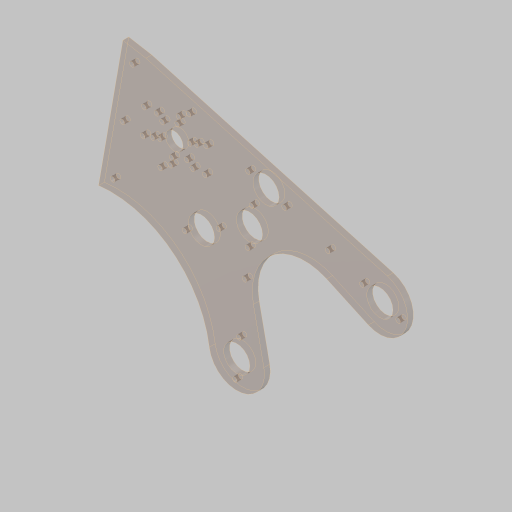
# Autodesk Inventor part: GP7-001
Saved by Autodesk Inventor 2023.5 (Build 275446000, 446)
## iProperties
Created: 2025-02-24
Part Number: GP7-001
Material: Polycarbonate, Smoke
Document SubType Name: Modeling
Designer: dlangdon
Density: 1.2 g/cm^3
Appearance: Polycarbonate - Smoked
Author: dlangdon
Autodesk Inventor part; units mm, degrees
ref_plane "YZ Plane" through (0, 0, 0) normal (1, 0, 0) x (0, 1, 0)
ref_plane "XZ Plane" through (0, 0, 0) normal (0, 1, 0) x (-1, 0, 0)
ref_plane "XY Plane" through (0, 0, 0) normal (0, 0, 1) x (1, 0, 0)
sketch "Sketch1" plane through (0, 0, 0) normal (0, 0, 1) x (1, 0, 0)
  circle A0 centre (77.8301, 65.3072) radius 50.8 construction
  circle A1 centre (-77.8301, -65.3072) radius 50.8 construction
  circle A2 centre (0, 0) radius 50.8 construction
  line L0 (-38.9151, -32.6536) -> (38.9151, 32.6536) construction
  line L1 (77.8301, 65.3072) -> (-77.8301, -65.3072) construction
  line L2 (-3.81, 6.5991) -> (-3.81, 50.6569) construction
  line L3 (-409.5487, -116.1072) -> (455.8434, -116.1072) construction
  circle A3 centre (141.8525, -58.9572) radius 57.15 construction
  circle A4 centre (77.8301, 65.3072) radius 14.2621
  circle A5 centre (-77.8301, -65.3072) radius 14.2621
  circle A6 centre (-3.81, 6.5991) radius 57.15 construction
  circle A7 centre (-77.8301, -65.3072) radius 30.1371 construction
  circle A8 centre (77.8301, 65.3072) radius 30.1371 construction
  circle A9 centre (-46.054, 109.6985) radius 14.2621
  line L4 (-46.054, 109.6985) -> (77.8301, 65.3072) construction
  circle A10 centre (77.8301, 65.3072) radius 14.2875 construction
  circle A11 centre (-77.8301, -65.3072) radius 14.2875 construction
  circle A12 centre (-64.0611, 65.5679) radius 14.2621
  line L5 (-77.8301, -65.3072) -> (-64.0611, 65.5679) construction
  circle A13 centre (-64.0611, 65.5679) radius 23.8316 construction
  circle A14 centre (-46.054, 109.6985) radius 23.8316 construction
  line L6 (19.8995, 58.5989) -> (65.3273, 37.886)
  line L7 (-48.3441, -59.0766) -> (-59.7253, -5.2163)
  arc A15 (19.8995, 58.5989) -> (-59.7253, -5.2163) centre (-3.81, 6.5991) ccw
  line L8 (-201.688, 172.6254) -> (-176.6739, 168.2148)
  line L9 (-176.6739, 168.2148) -> (-203.1379, 18.1301) construction
  line L10 (-203.1379, 18.1301) -> (-228.152, 22.5407) construction
  line L11 (-228.152, 22.5407) -> (-201.688, 172.6254) construction
  line L12 (-247.4634, -86.98) -> (29.0821, -135.7424) construction
  line L13 (-202.7907, 166.3719) -> (190.615, 97.0039) construction
  line L14 (-202.7907, 166.3719) -> (-247.4634, -86.98) construction
  circle A16 centre (-145.793, 105.6556) radius 31.75 construction
  line L15 (-66.5546, 41.8671) -> (-72.5149, -14.786) construction
  circle A17 centre (21.0409, 85.6565) radius 9.525 construction
  line L16 (-189.1809, 170.4201) -> (-215.6449, 20.3354) construction
  line L17 (-191.9376, 154.7863) -> (-212.8883, 35.9692) construction
  circle A18 centre (-145.793, 105.6556) radius 17.4625 construction
  circle A19 centre (-145.793, 105.6556) radius 9.525
  circle A20 centre (-46.054, 109.6985) radius 30.1816 construction
  line L18 (-201.688, 172.6254) -> (-228.152, 22.5407)
  arc A21 (65.3273, 37.886) -> (85.9918, 94.3181) centre (77.8301, 65.3072) ccw
  arc A22 (-107.6731, -69.5072) -> (-48.3441, -59.0766) centre (-77.8301, -65.3072) ccw
  line L19 (-145.793, 105.6556) -> (-129.3836, 111.6281) construction
  line L20 (-111.4825, 118.1436) -> (-180.1035, 93.1676) construction
  circle A23 centre (-180.1035, 93.1676) radius 4.7625 construction
  line L21 (0, 0) -> (-3.81, 6.5991) construction
  circle A24 centre (77.8301, 65.3072) radius 28.6512 construction
  line L22 (65.2741, 39.5538) -> (-52.3042, 96.8789) construction
  line L23 (84.4878, 93.1742) -> (-42.7399, 123.5703) construction
  line L24 (-176.6739, 168.2148) -> (85.9918, 94.3181)
  line L25 (-145.793, 105.6556) -> (-116.2701, 36.6349) construction
  circle A25 centre (-116.2701, 36.6349) radius 31.75 construction
  circle A26 centre (-116.2701, 36.6349) radius 14.2621
  line L26 (-64.0611, 65.5679) -> (-116.2701, 36.6349) construction
  circle A27 centre (-145.793, 105.6556) radius 25.4 construction
  arc A28 (-107.6731, -69.5072) -> (-228.152, 22.5407) centre (-214.5697, -84.5514) ccw
  circle A29 centre (-145.793, 105.6556) radius 36.5125 construction
  line L27 (-178.8846, 121.0865) -> (-145.793, 105.6556) construction
  point P0 (-69.5348, 13.5405)
  point P1 (-202.4129, 95.3778)
  point P2 (-202.4129, 95.3778)
  point P3 (-142.7607, 122.8528)
  point P4 (-159.1701, 116.8803)
  point P5 (-162.2024, 99.6831)
  point P6 (-148.8254, 88.4584)
  point P7 (-132.416, 94.4309)
  point P8 (-121.9248, 114.3429)
  point P9 (-141.3824, 130.6697)
  point P10 (-165.2505, 121.9824)
  point P11 (-169.6612, 96.9683)
  point P12 (-150.2037, 80.6415)
  point P13 (-126.3355, 89.3288)
  point P14 (-158.281, 139.9661)
  point P15 (-180.1035, 93.1676)
  point P16 (-133.305, 71.3451)
  point P17 (-130.3622, 138.7472)
  point P18 (-161.2239, 72.564)
  point P19 (-112.7015, 90.2248)
  dimension "d7" = 101.6
  dimension "d18" = 47.6631
  dimension "d34" = 34.925
  dimension "d65" = 50.8
  dimension "d3" = 50
  dimension "d4" = 0
  dimension "d8" = 101.6
  dimension "d9" = 28.5242
  dimension "d10" = 101.6
  dimension "d11" = 114.3
  dimension "d12" = 114.3
  dimension "d13" = 15.875
  dimension "d14" = 15.875
  dimension "d15" = 131.5974
  dimension "d16" = 28.575
  dimension "d17" = 131.5974
  dimension "d19" = 47.6631
  dimension "d22" = 25.4
  dimension "d23" = 152.4
  dimension "d26" = 257.2602
  dimension "d27" = 63.5
  dimension "d30" = 203.2
  dimension "d31" = 10
  dimension "d32" = 19.05
  dimension "d33" = 120.65
  dimension "d35" = 19.05
  dimension "d36" = 6.35
  dimension "d40" = 360
  dimension "d44" = 9.525
  dimension "d55" = 80
  dimension "d56" = 7.62
  dimension "d58" = 57.3024
  dimension "d59" = 63.5
  dimension "d60" = 75.0697
  dimension "d61" = 59.69
  dimension "d62" = 55
  dimension "d68" = 360
  dimension "d70" = 41.275
  dimension "d71" = 60
  dimension "d82" = 360
  dimension "d87" = 360
  dimension "d89" = 45
  dimension "d90" = 6.35
  dimension "d91" = 20.955
  dimension "d92" = 107.95
  constraints: 56 end point, 26 centre point, 24 coincident, 23 point on circle, 14 tangent, 7 midpoint, 6 equal radius, 5 point on line, 4 collinear, 4 parallel, 2 horizontal, 1 concentric, 1 perpendicular, 1 vertical, 39 other
  measures "d3" angle of L2 L0
  measures "d4" distance between parallel lines of L0 L1
  measures "d8" diameter of A2
  measures "d9" diameter of A4
  measures "d10" diameter of A0
  measures "d11" diameter of A3
  measures "d12" diameter of A6
  measures "d13" radial gap between concentric circles of A5 A7
  measures "d14" radial gap between concentric circles of A4 A8
  measures "d15" distance of L4.start L4.end
  measures "d16" diameter of A10
  measures "d17" distance of L5.start L5.end
  measures "d19" diameter of A14
  measures "d22" distance of L9.end L10.end
  measures "d23" distance of L10.end L8.start
  measures "d26" distance of L13.start L12.start
  measures "d27" diameter of A16
  measures "d30" distance from line of point (0, 0) L9
  measures "d31" angle of L3 L12
  measures "d32" diameter of A17
  measures "d33" distance of L17.start L17.end
  measures "d35" diameter of A19
  measures "d36" radial gap between concentric circles of A14 A20
  measures "d44" diameter of A23
  measures "d55" angle of L1 L21
  measures "d56" distance of L21.start L21.end
  measures "d58" diameter of A24
  measures "d59" diameter of A25
  measures "d60" distance of L19.start L25.end
  measures "d61" distance of L26.start L26.end
  measures "d62" angle of L15 L26
  measures "d70" distance from line of L9 L19.start
  measures "d71" angle of L9 L20
  measures "d89" angle of L20 L27
  measures "d90" distance between parallel lines of L8 L13
  measures "d91" distance from line of L24 L4.start
  measures "d92" radius of A28
extrude "Extrusion1" add sketch "Sketch1" along normal blind 6.35
hole "Hole1" at (21.0409, 85.6565, 0) at (-191.9376, 154.7863, 0) at (-202.4129, 95.3778, 0) at (-212.8883, 35.9692, 0) at (-129.3836, 111.6281, 0) at (-142.7607, 122.8528, 0) at (-159.1701, 116.8803, 0) at (-162.2024, 99.6831, 0) at (-148.8254, 88.4584, 0) at (-132.416, 94.4309, 0) at (-111.4825, 118.1436, 0) at (-180.1035, 93.1676, 0) at (-150.2037, 80.6415, 0) at (-169.6612, 96.9683, 0) at (-165.2505, 121.9824, 0) at (-141.3824, 130.6697, 0) at (-121.9248, 114.3429, 0) at (-126.3355, 89.3288, 0) at (-69.5348, 13.5405, 0) at (-178.8846, 121.0865, 0) at (-130.3622, 138.7472, 0) at (-112.7015, 90.2248, 0) at (-161.2239, 72.564, 0) direction (0, 0, 1) diameter 5.1054 end through all clearance for "Flat Head Machine Screw (82)" size "#10" standard "Ansi Unified Screw Threads"
sketch "Sketch2" plane through (0, 0, 6.35) normal (0, 0, 1) x (1, 0, 0)
  circle A0 centre (-126.3355, 89.3288) radius 2.5527 construction
  circle A1 centre (-141.3824, 130.6697) radius 2.5527 construction
  circle A2 centre (-169.6612, 96.9683) radius 2.5527 construction
  circle A3 centre (-180.1035, 93.1676) radius 2.5527 construction
  circle A4 centre (-132.416, 94.4309) radius 2.5527 construction
  circle A5 centre (-162.2024, 99.6831) radius 2.5527 construction
  circle A6 centre (-142.7607, 122.8528) radius 2.5527 construction
  circle A7 centre (-212.8883, 35.9692) radius 2.5527 construction
  circle A8 centre (-191.9376, 154.7863) radius 2.5527 construction
  circle A9 centre (21.0409, 85.6565) radius 2.5527 construction
  circle A10 centre (-202.4129, 95.3778) radius 2.5527 construction
  circle A11 centre (-129.3836, 111.6281) radius 2.5527 construction
  circle A12 centre (-159.1701, 116.8803) radius 2.5527 construction
  circle A13 centre (-148.8254, 88.4584) radius 2.5527 construction
  circle A14 centre (-111.4825, 118.1436) radius 2.5527 construction
  circle A15 centre (-150.2037, 80.6415) radius 2.5527 construction
  circle A16 centre (-165.2505, 121.9824) radius 2.5527 construction
  circle A17 centre (-121.9248, 114.3429) radius 2.5527 construction
  circle A18 centre (-69.5348, 13.5405) radius 2.5527 construction
  line L0 (-48.3441, -59.0766) -> (-59.7253, -5.2163) construction
  arc A19 (19.8995, 58.5989) -> (-59.7253, -5.2163) centre (-3.81, 6.5991) ccw construction
  line L1 (19.8995, 58.5989) -> (65.3273, 37.886) construction
  arc A20 (65.3273, 37.886) -> (85.9918, 94.3181) centre (77.8301, 65.3072) ccw construction
  line L2 (85.9918, 94.3181) -> (-176.6739, 168.2148) construction
  line L3 (-176.6739, 168.2148) -> (-201.688, 172.6254) construction
  line L4 (-201.688, 172.6254) -> (-228.152, 22.5407) construction
  arc A21 (-107.6731, -69.5072) -> (-228.152, 22.5407) centre (-214.5697, -84.5514) ccw construction
  arc A22 (-107.6731, -69.5072) -> (-48.3441, -59.0766) centre (-77.8301, -65.3072) ccw construction
  circle A23 centre (-64.0611, 65.5679) radius 14.2621 construction
  circle A24 centre (-145.793, 105.6556) radius 9.525 construction
  circle A25 centre (-116.2701, 36.6349) radius 14.2621 construction
  circle A26 centre (-46.054, 109.6985) radius 14.2621 construction
  circle A27 centre (-77.8301, -65.3072) radius 14.2621 construction
  circle A28 centre (77.8301, 65.3072) radius 14.2621 construction
  line L5 (-75.631, -44.4041) -> (-80.0293, -86.2104) construction
  line L6 (-134.6544, 26.4468) -> (-97.8859, 46.823) construction
  line L7 (-61.862, 86.471) -> (-66.2603, 44.6647) construction
  line L8 (-65.8406, 116.7886) -> (-26.2675, 102.6084) construction
  line L9 (58.0436, 72.3973) -> (97.6167, 58.2171) construction
  circle A29 centre (-64.0611, 65.5679) radius 14.2621 construction
  line L10 (-46.054, 109.6985) -> (-64.0611, 65.5679) construction
  line L11 (-46.054, 109.6985) -> (77.8301, 65.3072) construction
  line L12 (-64.0611, 65.5679) -> (-116.2701, 36.6349) construction
  line L13 (-64.0611, 65.5679) -> (-77.8301, -65.3072) construction
  circle A30 centre (-112.7015, 90.2248) radius 2.5527 projected
  point P0 (0, 0)
  point P1 (-116.0598, 70.5176)
  point P2 (-113.1961, 73.3575)
  dimension "d72" = 42.037
  constraints: 19 end point, 14 coincident, 5 collinear, 5 midpoint, 4 equal length, 1 other
  measures "d72" distance of L5.start L5.end
hole "Hole2" at (-75.631, -44.4041, 6.35) at (-97.8859, 46.823, 6.35) at (-80.0293, -86.2104, 6.35) at (-134.6544, 26.4468, 6.35) at (-66.2603, 44.6647, 6.35) at (-61.862, 86.471, 6.35) at (-26.2675, 102.6084, 6.35) at (-65.8406, 116.7886, 6.35) at (97.6167, 58.2171, 6.35) at (58.0436, 72.3973, 6.35) direction (0, 0, -1) diameter 5.1054 end through all clearance for "Flat Head Machine Screw (82)" size "#10" standard "Ansi Unified Screw Threads"
body "Solid1"
